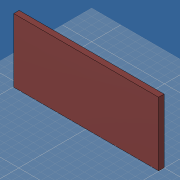
# Autodesk Inventor part: Front_Elektronik
Saved by Autodesk Inventor 2019 (Build 230136000, 136)
## iProperties
Created: 2020-08-05
Part Number: Front_Elektronik
Material: Generisch
Document SubType Name: Modeling
Designer: Stefan
Mass: 1372.35 g
Surface Area: 1626.58 cm^2
Volume: 1372.35 cm^3
Density: 1 g/cm^3
Appearance: Kastanie
Author: Stefan
Autodesk Inventor part; units mm, degrees
ref_plane "YZ Plane" through (0, 0, 0) normal (1, 0, 0) x (0, 1, 0)
ref_plane "XZ Plane" through (0, 0, 0) normal (0, 1, 0) x (-1, 0, 0)
ref_plane "XY Plane" through (0, 0, 0) normal (0, 0, 1) x (1, 0, 0)
sketch "Skizze1" plane through (0, 0, 0) normal (0, 0, 1) x (1, 0, 0)
  line L0 (199, -87.5) -> (-199, -87.5)
  line L1 (-199, -87.5) -> (-199, 87.5)
  line L2 (-199, 87.5) -> (199, 87.5)
  line L3 (199, 87.5) -> (199, -87.5)
  line L4 (199, -87.5) -> (-199, 87.5) construction
  line L5 (-199, -87.5) -> (199, 87.5) construction
  line L6 (-182, 70.5) -> (182, 70.5)
  line L7 (182, 70.5) -> (182, -79.5)
  line L8 (182, -79.5) -> (-182, -79.5)
  line L9 (-182, -79.5) -> (-182, 70.5)
  line L10 (-182, 70.5) -> (182, -79.5) construction
  line L11 (182, 70.5) -> (-182, -79.5) construction
  point P0 (0, 0)
  point P1 (0, -4.5)
  point P2 (0, -4.5)
  point P3 (0, 0)
  dimension "d0" = 175
  dimension "d1" = 398
  dimension "d2" = 8
  dimension "d3" = 17
  dimension "d4" = 17
  constraints: 24 end point, 6 midpoint, 4 parallel, 2 horizontal, 2 perpendicular, 1 vertical alignment
  measures "d0" distance of L0.end L1.end
  measures "d1" distance of L1.end L2.end
  measures "d2" distance between parallel lines of L0 L8
  measures "d3" distance between parallel lines of L2 L6
  measures "d4" distance between parallel lines of L9 L1
extrude "Extrusion1" add sketch "Skizze1" along normal blind 15 contours L0 L1 L2 L3 | L6 L7 L8 L9
extrude "Extrusion2" add sketch "Skizze1" against normal blind 6 contours L6 L7 L8 L9
equation "\"d1\" = case_width - 2 * gap_air"
equation "\"d5\" = inner_thickness"
equation "\"d7\" = mdf_thickness"
equation "\"kg_thickness\" = 4.9"
equation "\"ht_thickness\" = 1.9"
equation "\"case_thickness\" = 18"
equation "\"inner_thickness\" = 15"
equation "\"gap_fit\" = 0.1"
equation "\"gap_slide\" = 0.2"
equation "\"gap_air\" = 1"
equation "\"bore_diameter\" = 73"
equation "\"mdf_thickness\" = 6"
equation "\"tape_width\" = 15"
equation "\"tape_thickness\" = 3"
equation "\"inner_depth\" = 255"
equation "\"case_width\" = 400"
